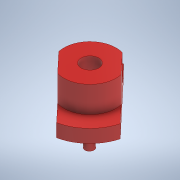
# Autodesk Inventor part: Adaptation_on_OPdevside_4_3
Saved by Autodesk Inventor 2022 (Build 260153000, 153)
## iProperties
Created: 2021-10-05
Part Number: Adaptation_on_OPdevside_4_3
Material: Generisch
Document SubType Name: Modeling
Designer: 123St
Density: 1 g/cm^3
Appearance: Orangerot
Author: 123St
Autodesk Inventor part; units mm, degrees
ref_plane "YZ Plane" through (0, 0, 0) normal (1, 0, 0) x (0, 1, 0)
ref_plane "XZ Plane" through (0, 0, 0) normal (0, 1, 0) x (-1, 0, 0)
ref_plane "XY Plane" through (0, 0, 0) normal (0, 0, 1) x (1, 0, 0)
sketch "Skizze1" plane through (0, 0, 0) normal (0, 1, 0) x (-1, 0, 0)
  circle A0 centre (0, 0) radius 15
  dimension "d0" = 30
  constraints: 1 centre point, 1 coincident
  measures "d0" diameter of A0
extrude "Extrusion1" add sketch "Skizze1" along normal blind 10
sketch "Skizze2" plane through (0, 0, 0) normal (0, -1, 0) x (1, 0, 0)
  line L0 (14.3188, 0.9) -> (12.9688, 0.9)
  line L1 (12.9688, -0.9) -> (14.3188, -0.9)
  line L2 (14.3188, -0.9) -> (14.3188, 0.9)
  line L3 (-21.3175, 0) -> (21.3175, 0) projected
  arc A0 (12.9688, 0.9) -> (0.9, 12.9688) centre (0, 0) ccw
  line L4 (-0.9, -12.9688) -> (-0.9, -14.3188)
  line L5 (-0.9, -14.3188) -> (0.9, -14.3188)
  line L6 (0.9, -14.3188) -> (0.9, -12.9688)
  line L7 (-12.9688, 0.9) -> (-14.3188, 0.9)
  line L8 (-14.3188, 0.9) -> (-14.3188, -0.9)
  line L9 (-14.3188, -0.9) -> (-12.9688, -0.9)
  line L10 (-0.9, 12.9688) -> (-0.9, 14.3188)
  line L11 (-0.9, 14.3188) -> (0.9, 14.3188)
  line L12 (0.9, 14.3188) -> (0.9, 12.9688)
  line L13 (0, -21.3175) -> (0, 21.3175) projected
  line L14 (-21.3175, 0) -> (21.3175, 0) projected
  arc A1 (0.9, -12.9688) -> (12.9688, -0.9) centre (0, 0) ccw
  arc A2 (-12.9688, -0.9) -> (-0.9, -12.9688) centre (0, 0) ccw
  arc A3 (-0.9, 12.9688) -> (-12.9688, 0.9) centre (0, 0) ccw
  circle A4 centre (0, 0) radius 4.2
  circle A5 centre (7, 7.1414) radius 1.2
  circle A6 centre (-5.6, -5.7131) radius 1.2
  dimension "d4" = 0.9
  dimension "d5" = 0.9
  dimension "d8" = 1.35
  dimension "d9" = 1.35
  dimension "d10" = 1.8
  dimension "d11" = 0.9
  dimension "d12" = 1.35
  dimension "d13" = 1.8
  dimension "d14" = 0.9
  dimension "d15" = 0.9
  dimension "d16" = 1.35
  dimension "d17" = 8.4
  dimension "d18" = 2.4
  dimension "d19" = 2.4
  dimension "d20" = 8
  dimension "d21" = 10
  dimension "d22" = 7
  dimension "d23" = 5.6
  dimension "d50" = 13
  dimension "d51" = 13
  dimension "d52" = 1.35
  dimension "d53" = 1.35
  dimension "d54" = 1.35
  constraints: 24 end point, 10 point on circle, 7 centre point, 5 coincident, 4 parallel, 2 horizontal, 1 perpendicular, 1 point on line
  measures "d4" distance between parallel lines of L3 L1
  measures "d5" distance between parallel lines of L3 L0
  measures "d8" distance of L1.start L1.end
  measures "d9" distance of L5.end L6.end
  measures "d10" distance of L4.end L5.end
  measures "d11" distance between parallel lines of L4 L13
  measures "d12" distance of L8.end L9.end
  measures "d13" distance of L7.end L8.end
  measures "d14" distance between parallel lines of L14 L7
  measures "d15" distance between parallel lines of L13 L12
  measures "d16" distance of L11.end L12.end
  measures "d17" diameter of A4
  measures "d18" diameter of A5
  measures "d19" diameter of A6
  measures "d20" distance of point (0, 0) A6.centre
  measures "d21" distance of point (0, 0) A5.centre
  measures "d22" distance from line of L13 A5.centre
  measures "d23" distance from line of A6.centre L13
  measures "d50" radius of A1
  measures "d51" radius of A2
  measures "d52" distance of L4.start L4.end
  measures "d53" distance of L0.start L0.end
  measures "d54" distance of L10.start L10.end
extrude "Extrusion2" cut sketch "Skizze2" against normal blind 3 contours L2 L3 A4 L13 L11 L12 A0 L0 | L2 L1 A1 L6 L5 L13 A4 L3 | A4 L3 L8 L7 A3 L10 L11 L13 | L13 L5 L4 A2 L9 L8 L3 A4
sketch "Skizze4" plane through (7, 0, 7.1414) normal (0, -1, 0) x (1, 0, 0)
  circle A0 centre (-7, -7.1414) radius 4.2
  circle A1 centre (-12.6, -12.8546) radius 1.2
  circle A2 centre (0, 0) radius 1.2
  line L0 (-7, -28.1414) -> (-7, 13.8586) projected
  dimension "d26" = 2.4
  dimension "d27" = 5.6
  dimension "d28" = 8
  dimension "d44" = 8.4
  dimension "d45" = 2.4
  constraints: 3 centre point, 1 coincident
  measures "d26" diameter of A1
  measures "d27" distance from line of L0 A1.centre
  measures "d28" distance of A1.centre point (-7, -7.141)
  measures "d44" diameter of A0
  measures "d45" diameter of A2
extrude "Extrusion3" add sketch "Skizze4" along normal blind 2
sketch "Skizze5" plane through (0, 10, 0) normal (0, 1, 0) x (1, 0, 0)
  circle A0 centre (0, 0) radius 19.262
  circle A1 centre (0, 0) radius 7
  dimension "d31" = 14
  constraints: 2 centre point, 2 coincident
  measures "d31" diameter of A1
extrude "Extrusion4" cut sketch "Skizze5" against normal blind 7
fillet "Rundung1" radius 1 8 edges at (12.9688, 1.5, -0.9) (12.9688, 1.5, 0.9) (0.9, 1.5, -12.9688) (-0.9, 1.5, -12.9688) (-12.9688, 1.5, -0.9) (-12.9688, 1.5, 0.9) (-0.9, 1.5, 12.9688) (0.9, 1.5, 12.9688)
sketch "Skizze8" plane through (0, 10, 0) normal (0, 1, 0) x (1, 0, 0)
  circle A0 centre (0, 0) radius 1
  dimension "d46" = 2
  constraints: 1 centre point, 1 coincident
  measures "d46" diameter of A0
extrude "Extrusion7" cut sketch "Skizze8" against normal blind 7
sketch "Skizze9" plane through (0, -2, 0) normal (0, -1, 0) x (1, 0, 0)
  line L0 (18.2687, 9.2162) -> (-7.478, -18.1772)
  line L1 (-7.478, -18.1772) -> (18.2687, -18.1772)
  line L2 (18.2687, -18.1772) -> (18.2687, 9.2162)
  line L3 (8.0673, 18.8043) -> (-17.6793, -8.5891)
  line L4 (-17.6793, -8.5891) -> (-17.6793, 18.8043)
  line L5 (-17.6793, 18.8043) -> (8.0673, 18.8043)
  point P0 (0, 0)
  dimension "d55" = 7
  dimension "d56" = 7
  constraints: 12 end point, 2 parallel, 2 perpendicular, 1 horizontal
  measures "d55" distance from line of L0 point (0, 0)
  measures "d56" distance from line of point (0, 0) L3
extrude "Extrusion8" cut sketch "Skizze9" against normal blind 50
sketch "Skizze10" plane through (0, -2, 0) normal (0, -1, 0) x (1, 0, 0)
  circle A0 centre (0, 0) radius 11.5
  circle A1 centre (0, 0) radius 18.9246
  dimension "d61" = 23
  constraints: 2 centre point, 2 coincident
  measures "d61" diameter of A0
extrude "Extrusion9" cut sketch "Skizze10" against normal blind 10
sketch "Skizze11" plane through (0, -2, 0) normal (0, -1, 0) x (1, 0, 0)
  circle A0 centre (0, 0) radius 1 projected
  circle A1 centre (0, 0) radius 4.2
  constraints: 1 centre point, 1 coincident
extrude "Extrusion10" cut sketch "Skizze11" against normal blind 8.5 contours A0 | A1
sketch "Skizze13" plane through (0, 3, 0) normal (0, -1, 0) x (1, 0, 0)
  circle A0 centre (7, 7.1414) radius 1.2 projected
  circle A1 centre (7, 7.1414) radius 1.2
  circle A2 centre (-5.6, -5.7131) radius 1.2 projected
  circle A3 centre (-5.6, -5.7131) radius 1.2
  arc A4 (11.3495, 1.8544) -> (1.1481, 11.4425) centre (0, 0) ccw
  line L0 (11.3495, 1.8544) -> (8.9749, -0.6721) projected
  line L1 (11.3495, 1.8544) -> (-1.1481, -11.4425)
  line L2 (1.1481, 11.4425) -> (-11.3495, -1.8544)
  line L3 (1.2265, -8.916) -> (-1.1481, -11.4425) projected
  arc A5 (-11.3495, -1.8544) -> (-1.1481, -11.4425) centre (0, 0) ccw
  circle A6 centre (0, 0) radius 4.2
  constraints: 5 centre point, 5 point on circle, 4 coincident, 4 end point, 1 collinear, 3 other
extrude "Extrusion11" add sketch "Skizze13" along normal blind 3.5
sketch "Skizze14" plane through (7, -2, 7.1414) normal (0, -1, 0) x (1, 0, 0)
  circle A0 centre (0, 0) radius 1.2 projected
  circle A1 centre (0, 0) radius 1.2
  circle A2 centre (-12.6, -12.8546) radius 1.2 projected
  circle A3 centre (-12.6, -12.8546) radius 1.2
  point P0 (-7, -7.1414)
  constraints: 2 centre point, 2 coincident
extrude "Extrusion12" add sketch "Skizze14" along normal blind 0.5
sketch "Skizze15" plane through (0, 10, 0) normal (0, 1, 0) x (1, 0, 0)
  circle A0 centre (0, 0) radius 1 projected
  circle A1 centre (0, 0) radius 2.35
  dimension "d68" = 4.7
  constraints: 1 centre point, 1 coincident
  measures "d68" diameter of A1
extrude "Extrusion13" cut sketch "Skizze15" against normal blind 3.3 contours A0 | A1
sketch "Skizze17" plane through (0, -0.5, 0) normal (0, -1, 0) x (1, 0, 0)
  line L0 (2.8954, 11.8415) -> (-13.3125, -5.4031)
  line L1 (1.1481, 11.4425) -> (-5.1007, 4.7941) projected
  line L2 (-13.3125, -5.4031) -> (-13.3125, 19.7684)
  line L3 (-13.3125, 19.7684) -> (2.8954, 11.8415)
  line L4 (-3.5303, -12.5169) -> (12.8557, 4.9171)
  line L5 (-1.1481, -11.4425) -> (5.1007, -4.7941) projected
  line L6 (12.8557, 4.9171) -> (12.8557, -12.5169)
  line L7 (12.8557, -12.5169) -> (-3.5303, -12.5169)
  point P0 (0, 0)
  dimension "d71" = 1
  dimension "d72" = 1
  constraints: 12 end point, 3 parallel, 1 perpendicular, 1 vertical
  measures "d71" distance between parallel lines of L1 L0
  measures "d72" distance between parallel lines of L5 L4
extrude "Extrusion14" cut sketch "Skizze17" against normal blind 15
